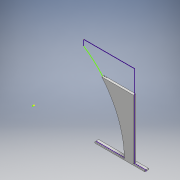
# Autodesk Inventor part: mtv_angle_2-2
Saved by Autodesk Inventor 2018 (Build 220112000, 112)
## iProperties
Created: 2019-02-03
Part Number: mtv_angle_2-2
Material: Generic
Document SubType Name: Modeling
Designer: Aditya Kendre
Density: 1 g/cm^3
Appearance: Default
Author: Aditya Kendre
## iProperties of the stored document mtv_angle_2-2_3DPrint.ipt
Created: 2019-02-03
Part Number: mtv_angle_2-2_3DPrint
Material: Generic
Document SubType Name: Modeling
Designer: Aditya Kendre
Density: 1 g/cm^3
Appearance: Default
Author: Aditya Kendre
Autodesk Inventor part; units mm, degrees
(part 1 of 2)
ref_plane "YZ Plane" through (0, 0, 0) normal (1, 0, 0) x (0, 1, 0)
ref_plane "XZ Plane" through (0, 0, 0) normal (0, 1, 0) x (-1, 0, 0)
ref_plane "XY Plane" through (0, 0, 0) normal (0, 0, 1) x (1, 0, 0)
sketch "Sketch1" plane through (0, 0, 0) normal (0, 1, 0) x (-1, 0, 0)
  line L0 (-225, -225) -> (225, -225)
  line L1 (225, -225) -> (225, 225)
  line L2 (225, 225) -> (-225, 225)
  line L3 (-225, 225) -> (-225, -225)
  line L4 (-225, -225) -> (225, 225) construction
  line L5 (225, -225) -> (-225, 225) construction
  point P0 (0, 0)
  dimension "d0" = 450
  dimension "d1" = 450
  constraints: 12 end point, 2 midpoint, 2 parallel, 1 horizontal, 1 perpendicular
  measures "d0" distance of L2.end L1.end
  measures "d1" distance of L1.end L0.end
extrude "Extrusion1" add sketch "Sketch1" along normal blind 3
sketch "Sketch2" plane through (0, 3, 0) normal (0, 1, 0) x (1, 0, 0)
  circle A0 centre (0, 0) radius 205
  dimension "d4" = 410
  constraints: 1 centre point, 1 coincident
  measures "d4" diameter of A0
extrude "Extrusion2" cut sketch "Sketch2" against normal blind 3
sketch "Sketch3" plane through (0, 3, 0) normal (0, 1, 0) x (1, 0, 0)
  circle A0 centre (0, 0) radius 205 projected
  line L0 (205, 0) -> (225, 0)
  line L1 (225, -225) -> (225, 225) projected
  line L2 (225, 0) -> (225, -225)
  line L3 (225, -225) -> (112.5, -225)
  line L4 (-225, -225) -> (225, -225) projected
  line L5 (112.5, -225) -> (112.5, 0)
  line L6 (112.5, 0) -> (225, 0)
  line L7 (112.5, -225) -> (-258.9889, -225)
  line L8 (-258.9889, -225) -> (-258.9889, 323.9574)
  line L9 (-258.9889, 323.9574) -> (112.5, 323.9574)
  line L10 (112.5, 323.9574) -> (112.5, -225)
  line L11 (225, 0) -> (-258.9889, 0)
  line L12 (-258.9889, 0) -> (-258.9889, 355.1924)
  line L13 (-258.9889, 355.1924) -> (225, 355.1924)
  line L14 (225, 355.1924) -> (225, 0)
  dimension "d7" = 112.5
  constraints: 26 end point, 4 parallel, 4 perpendicular, 3 point on line, 2 horizontal, 1 collinear, 1 horizontal alignment, 1 midpoint, 1 other
  measures "d7" distance of L1.start L3.end
extrude "Extrusion3" cut sketch "Sketch3" against normal blind 3 contours L6 L10 A0 | A0 L10 L9 L12 L13 L14 L1 L0 | L10 L11 A0 | A0 L11 L8 L9 L10 | L5 L4 L7 L8 L11 A0 | A0 L11 L5
sketch "Sketch4" plane through (0, 3, 0) normal (0, 1, 0) x (1, 0, 0)
  line L0 (112.5, -225) -> (225, -225) projected
  line L1 (225, -225) -> (225, 0) projected
  line L2 (112.5, -225) -> (225, -225)
  line L3 (225, -225) -> (225, -184.2834)
  line L4 (225, -184.2834) -> (112.5, -184.2834)
  line L5 (112.5, -184.2834) -> (112.5, -225)
  point P0 (0, 0)
  constraints: 8 end point, 2 parallel, 1 horizontal, 1 perpendicular, 1 point on line
extrude "Extrusion4" cut sketch "Sketch4" against normal blind 3
sketch "Sketch5" plane through (0, 3, 0) normal (0, 1, 0) x (1, 0, 0)
  line L0 (225, -184.2834) -> (225, 0) projected
  line L1 (225, 0) -> (140, 0)
  line L2 (140, 0) -> (140, -3)
  line L3 (140, -3) -> (225, -3)
  line L4 (225, -3) -> (225, 0)
  point P0 (0, 0)
  dimension "d12" = 85
  dimension "d13" = 3
  constraints: 8 end point, 2 parallel, 1 horizontal, 1 perpendicular
  measures "d12" distance of L3.end L2.end
  measures "d13" distance of L2.end L1.end
extrude "Extrusion5" add sketch "Sketch5" along normal mid plane 6
sketch "Sketch6" plane through (225, 0, 184.2834) normal (1, 0, 0) x (0, 0, -1)
  line L0 (181.2834, 3) -> (181.2834, 6) projected
  line L1 (184.2834, 0) -> (184.2834, 6) projected
  line L2 (181.2834, 6) -> (184.2834, 6)
  line L3 (184.2834, 6) -> (184.2834, 0)
  line L4 (184.2834, 0) -> (181.2834, 0)
  line L5 (181.2834, 0) -> (181.2834, 6)
  constraints: 8 end point, 2 parallel, 1 horizontal, 1 perpendicular
extrude "Extrusion6" add sketch "Sketch6" along normal blind 25
sketch "Sketch7" plane through (0, 3, 0) normal (0, 1, 0) x (1, 0, 0)
  arc A0 (112.5, -171.3731) -> (204.978, -3) centre (0, 0) ccw projected
  line L0 (204.978, -3) -> (140, -3) projected
  arc A1 (204.978, -3) -> (204.978, -3) centre (0, 0) ccw
  line L1 (112.5, -171.3731) -> (112.5, -173.3731)
  line L2 (112.5, -171.3731) -> (112.5, -184.2834) projected
  line L3 (204.978, -3) -> (206.978, -3)
  line L4 (140, -3) -> (250, -3) projected
  arc A2 (112.5, -173.3731) -> (206.978, -3) centre (3.682, -1.6473) ccw
  line L5 (206.1666, -3.9622) -> (206.1702, -3.6213)
  line L6 (206.1702, -3.6213) -> (210.1566, -3.6636)
  line L7 (210.1566, -3.6636) -> (210.153, -4.0044)
  line L8 (210.153, -4.0044) -> (206.1666, -3.9622)
  line L9 (206.1127, -6.8623) -> (206.1212, -6.5215)
  line L10 (206.1212, -6.5215) -> (210.1066, -6.6209)
  line L11 (210.1066, -6.6209) -> (210.0981, -6.9616)
  line L12 (210.0981, -6.9616) -> (206.1127, -6.8623)
  line L13 (206.0172, -9.7613) -> (206.0306, -9.4207)
  line L14 (206.0306, -9.4207) -> (210.0141, -9.5771)
  line L15 (210.0141, -9.5771) -> (210.0008, -9.9177)
  line L16 (210.0008, -9.9177) -> (206.0172, -9.7613)
  line L17 (205.8803, -12.6587) -> (205.8985, -12.3183)
  line L18 (205.8985, -12.3183) -> (209.8794, -12.5318)
  line L19 (209.8794, -12.5318) -> (209.8611, -12.8722)
  line L20 (209.8611, -12.8722) -> (205.8803, -12.6587)
  line L21 (205.7018, -15.5538) -> (205.7249, -15.2137)
  line L22 (205.7249, -15.2137) -> (209.7023, -15.4842)
  line L23 (209.7023, -15.4842) -> (209.6792, -15.8243)
  line L24 (209.6792, -15.8243) -> (205.7018, -15.5538)
  line L25 (205.4819, -18.4461) -> (205.5099, -18.1064)
  line L26 (205.5099, -18.1064) -> (209.483, -18.4338)
  line L27 (209.483, -18.4338) -> (209.455, -18.7735)
  line L28 (209.455, -18.7735) -> (205.4819, -18.4461)
  line L29 (205.2205, -21.3349) -> (205.2534, -20.9956)
  line L30 (205.2534, -20.9956) -> (209.2214, -21.3799)
  line L31 (209.2214, -21.3799) -> (209.1886, -21.7192)
  line L32 (209.1886, -21.7192) -> (205.2205, -21.3349)
  line L33 (204.9179, -24.2197) -> (204.9556, -23.8809)
  line L34 (204.9556, -23.8809) -> (208.9177, -24.322)
  line L35 (208.9177, -24.322) -> (208.88, -24.6608)
  line L36 (208.88, -24.6608) -> (204.9179, -24.2197)
  line L37 (204.5739, -27.0998) -> (204.6165, -26.7616)
  line L38 (204.6165, -26.7616) -> (208.5719, -27.2594)
  line L39 (208.5719, -27.2594) -> (208.5293, -27.5976)
  line L40 (208.5293, -27.5976) -> (204.5739, -27.0998)
  line L41 (204.1887, -29.9747) -> (204.2361, -29.6372)
  line L42 (204.2361, -29.6372) -> (208.184, -30.1916)
  line L43 (208.184, -30.1916) -> (208.1366, -30.5291)
  line L44 (208.1366, -30.5291) -> (204.1887, -29.9747)
  line L45 (203.7624, -32.8439) -> (203.8146, -32.507)
  line L46 (203.8146, -32.507) -> (207.7541, -33.1179)
  line L47 (207.7541, -33.1179) -> (207.7019, -33.4547)
  line L48 (207.7019, -33.4547) -> (203.7624, -32.8439)
  line L49 (203.295, -35.7066) -> (203.3521, -35.3705)
  line L50 (203.3521, -35.3705) -> (207.2824, -36.0378)
  line L51 (207.2824, -36.0378) -> (207.2254, -36.3738)
  line L52 (207.2254, -36.3738) -> (203.295, -35.7066)
  line L53 (202.7867, -38.5623) -> (202.8485, -38.2271)
  line L54 (202.8485, -38.2271) -> (206.7689, -38.9506)
  line L55 (206.7689, -38.9506) -> (206.7071, -39.2858)
  line L56 (206.7071, -39.2858) -> (202.7867, -38.5623)
  line L57 (202.2375, -41.4104) -> (202.3041, -41.0762)
  line L58 (202.3041, -41.0762) -> (206.2138, -41.8557)
  line L59 (206.2138, -41.8557) -> (206.1471, -42.19)
  line L60 (206.1471, -42.19) -> (202.2375, -41.4104)
  line L61 (201.6476, -44.2504) -> (201.719, -43.9171)
  line L62 (201.719, -43.9171) -> (205.6171, -44.7526)
  line L63 (205.6171, -44.7526) -> (205.5456, -45.0859)
  line L64 (205.5456, -45.0859) -> (201.6476, -44.2504)
  line L65 (201.017, -47.0817) -> (201.0932, -46.7494)
  line L66 (201.0932, -46.7494) -> (204.9789, -47.6407)
  line L67 (204.9789, -47.6407) -> (204.9027, -47.9729)
  line L68 (204.9027, -47.9729) -> (201.017, -47.0817)
  line L69 (200.346, -49.9036) -> (200.4269, -49.5725)
  line L70 (200.4269, -49.5725) -> (204.2995, -50.5193)
  line L71 (204.2995, -50.5193) -> (204.2185, -50.8504)
  line L72 (204.2185, -50.8504) -> (200.346, -49.9036)
  line L73 (199.6346, -52.7156) -> (199.7203, -52.3857)
  line L74 (199.7203, -52.3857) -> (203.5789, -53.3879)
  line L75 (203.5789, -53.3879) -> (203.4932, -53.7178)
  line L76 (203.4932, -53.7178) -> (199.6346, -52.7156)
  line L77 (198.883, -55.5172) -> (198.9734, -55.1885)
  line L78 (198.9734, -55.1885) -> (202.8172, -56.2459)
  line L79 (202.8172, -56.2459) -> (202.7268, -56.5745)
  line L80 (202.7268, -56.5745) -> (198.883, -55.5172)
  line L81 (198.0913, -58.3077) -> (198.1864, -57.9803)
  line L82 (198.1864, -57.9803) -> (202.0147, -59.0926)
  line L83 (202.0147, -59.0926) -> (201.9196, -59.42)
  line L84 (201.9196, -59.42) -> (198.0913, -58.3077)
  line L85 (197.2598, -61.0865) -> (197.3596, -60.7606)
  line L86 (197.3596, -60.7606) -> (201.1716, -61.9276)
  line L87 (201.1716, -61.9276) -> (201.0718, -62.2535)
  line L88 (201.0718, -62.2535) -> (197.2598, -61.0865)
  line L89 (196.3885, -63.8532) -> (196.493, -63.5287)
  line L90 (196.493, -63.5287) -> (200.2879, -64.7502)
  line L91 (200.2879, -64.7502) -> (200.1834, -65.0747)
  line L92 (200.1834, -65.0747) -> (196.3885, -63.8532)
  line L93 (195.4778, -66.6071) -> (195.5868, -66.2842)
  line L94 (195.5868, -66.2842) -> (199.3638, -67.5599)
  line L95 (199.3638, -67.5599) -> (199.2547, -67.8828)
  line L96 (199.2547, -67.8828) -> (195.4778, -66.6071)
  line L97 (194.5276, -69.3477) -> (194.6413, -69.0264)
  line L98 (194.6413, -69.0264) -> (198.3996, -70.356)
  line L99 (198.3996, -70.356) -> (198.2859, -70.6774)
  line L100 (198.2859, -70.6774) -> (194.5276, -69.3477)
  line L101 (193.5383, -72.0744) -> (193.6566, -71.7547)
  line L102 (193.6566, -71.7547) -> (197.3955, -73.1381)
  line L103 (197.3955, -73.1381) -> (197.2772, -73.4578)
  line L104 (197.2772, -73.4578) -> (193.5383, -72.0744)
  line L105 (192.51, -74.7866) -> (192.6329, -74.4687)
  line L106 (192.6329, -74.4687) -> (196.3516, -75.9055)
  line L107 (196.3516, -75.9055) -> (196.2287, -76.2234)
  line L108 (196.2287, -76.2234) -> (192.51, -74.7866)
  line L109 (191.443, -77.4839) -> (191.5704, -77.1677)
  line L110 (191.5704, -77.1677) -> (195.2681, -78.6576)
  line L111 (195.2681, -78.6576) -> (195.1408, -78.9738)
  line L112 (195.1408, -78.9738) -> (191.443, -77.4839)
  line L113 (190.3375, -80.1655) -> (190.4694, -79.8512)
  line L114 (190.4694, -79.8512) -> (194.1454, -81.394)
  line L115 (194.1454, -81.394) -> (194.0135, -81.7083)
  line L116 (194.0135, -81.7083) -> (190.3375, -80.1655)
  line L117 (189.1937, -82.8311) -> (189.3301, -82.5187)
  line L118 (189.3301, -82.5187) -> (192.9836, -84.1139)
  line L119 (192.9836, -84.1139) -> (192.8472, -84.4263)
  line L120 (192.8472, -84.4263) -> (189.1937, -82.8311)
  line L121 (188.0118, -85.48) -> (188.1526, -85.1696)
  line L122 (188.1526, -85.1696) -> (191.7829, -86.817)
  line L123 (191.7829, -86.817) -> (191.6421, -87.1274)
  line L124 (191.6421, -87.1274) -> (188.0118, -85.48)
  line L125 (186.7921, -88.1117) -> (186.9374, -87.8034)
  line L126 (186.9374, -87.8034) -> (190.5437, -89.5026)
  line L127 (190.5437, -89.5026) -> (190.3984, -89.8109)
  line L128 (190.3984, -89.8109) -> (186.7921, -88.1117)
  line L129 (185.5348, -90.7257) -> (185.6845, -90.4194)
  line L130 (185.6845, -90.4194) -> (189.2661, -92.1701)
  line L131 (189.2661, -92.1701) -> (189.1164, -92.4764)
  line L132 (189.1164, -92.4764) -> (185.5348, -90.7257)
  line L133 (184.2402, -93.3213) -> (184.3942, -93.0173)
  line L134 (184.3942, -93.0173) -> (187.9504, -94.8191)
  line L135 (187.9504, -94.8191) -> (187.7964, -95.1232)
  line L136 (187.7964, -95.1232) -> (184.2402, -93.3213)
  line L137 (182.9085, -95.8982) -> (183.0669, -95.5964)
  line L138 (183.0669, -95.5964) -> (186.597, -97.449)
  line L139 (186.597, -97.449) -> (186.4386, -97.7508)
  line L140 (186.4386, -97.7508) -> (182.9085, -95.8982)
  line L141 (181.5401, -98.4558) -> (181.7028, -98.1562)
  line L142 (181.7028, -98.1562) -> (185.2059, -100.0592)
  line L143 (185.2059, -100.0592) -> (185.0432, -100.3587)
  line L144 (185.0432, -100.3587) -> (181.5401, -98.4558)
  line L145 (180.1352, -100.9934) -> (180.3022, -100.6963)
  line L146 (180.3022, -100.6963) -> (183.7777, -102.6492)
  line L147 (183.7777, -102.6492) -> (183.6107, -102.9464)
  line L148 (183.6107, -102.9464) -> (180.1352, -100.9934)
  line L149 (178.6941, -103.5107) -> (178.8653, -103.216)
  line L150 (178.8653, -103.216) -> (182.3125, -105.2185)
  line L151 (182.3125, -105.2185) -> (182.1413, -105.5132)
  line L152 (182.1413, -105.5132) -> (178.6941, -103.5107)
  line L153 (177.2171, -106.0071) -> (177.3925, -105.7149)
  line L154 (177.3925, -105.7149) -> (180.8106, -107.7665)
  line L155 (180.8106, -107.7665) -> (180.6352, -108.0588)
  line L156 (180.6352, -108.0588) -> (177.2171, -106.0071)
  line L157 (175.7044, -108.4821) -> (175.884, -108.1924)
  line L158 (175.884, -108.1924) -> (179.2724, -110.2928)
  line L159 (179.2724, -110.2928) -> (179.0928, -110.5825)
  line L160 (179.0928, -110.5825) -> (175.7044, -108.4821)
  line L161 (174.1565, -110.9351) -> (174.3402, -110.648)
  line L162 (174.3402, -110.648) -> (177.6982, -112.7968)
  line L163 (177.6982, -112.7968) -> (177.5145, -113.0839)
  line L164 (177.5145, -113.0839) -> (174.1565, -110.9351)
  line L165 (172.5736, -113.3658) -> (172.7614, -113.0813)
  line L166 (172.7614, -113.0813) -> (176.0883, -115.278)
  line L167 (176.0883, -115.278) -> (175.9004, -115.5624)
  line L168 (175.9004, -115.5624) -> (172.5736, -113.3658)
  line L169 (170.956, -115.7735) -> (171.1479, -115.4917)
  line L170 (171.1479, -115.4917) -> (174.4429, -117.7358)
  line L171 (174.4429, -117.7358) -> (174.2511, -118.0175)
  line L172 (174.2511, -118.0175) -> (170.956, -115.7735)
  line L173 (169.3042, -118.1578) -> (169.5001, -117.8788)
  line L174 (169.5001, -117.8788) -> (172.7626, -120.1698)
  line L175 (172.7626, -120.1698) -> (172.5667, -120.4488)
  line L176 (172.5667, -120.4488) -> (169.3042, -118.1578)
  line L177 (167.6183, -120.5182) -> (167.8182, -120.242)
  line L178 (167.8182, -120.242) -> (171.0476, -122.5796)
  line L179 (171.0476, -122.5796) -> (170.8477, -122.8557)
  line L180 (170.8477, -122.8557) -> (167.6183, -120.5182)
  line L181 (165.8988, -122.8542) -> (166.1026, -122.5809)
  line L182 (166.1026, -122.5809) -> (169.2982, -124.9645)
  line L183 (169.2982, -124.9645) -> (169.0944, -125.2377)
  line L184 (169.0944, -125.2377) -> (165.8988, -122.8542)
  line L185 (164.146, -125.1653) -> (164.3537, -124.895)
  line L186 (164.3537, -124.895) -> (167.5148, -127.3241)
  line L187 (167.5148, -127.3241) -> (167.3071, -127.5944)
  line L188 (167.3071, -127.5944) -> (164.146, -125.1653)
  line L189 (162.3603, -127.4511) -> (162.5718, -127.1838)
  line L190 (162.5718, -127.1838) -> (165.6978, -129.6579)
  line L191 (165.6978, -129.6579) -> (165.4863, -129.9252)
  line L192 (165.4863, -129.9252) -> (162.3603, -127.4511)
  line L193 (160.542, -129.711) -> (160.7574, -129.4468)
  line L194 (160.7574, -129.4468) -> (163.8476, -131.9654)
  line L195 (163.8476, -131.9654) -> (163.6323, -132.2297)
  line L196 (163.6323, -132.2297) -> (160.542, -129.711)
  line L197 (158.6916, -131.9447) -> (158.9107, -131.6836)
  line L198 (158.9107, -131.6836) -> (161.9645, -134.2462)
  line L199 (161.9645, -134.2462) -> (161.7454, -134.5074)
  line L200 (161.7454, -134.5074) -> (158.6916, -131.9447)
  line L201 (156.8093, -134.1517) -> (157.0322, -133.8937)
  line L202 (157.0322, -133.8937) -> (160.049, -136.4999)
  line L203 (160.049, -136.4999) -> (159.8261, -136.7578)
  line L204 (159.8261, -136.7578) -> (156.8093, -134.1517)
  line L205 (154.8957, -136.3315) -> (155.1222, -136.0767)
  line L206 (155.1222, -136.0767) -> (158.1013, -138.7258)
  line L207 (158.1013, -138.7258) -> (157.8748, -138.9805)
  line L208 (157.8748, -138.9805) -> (154.8957, -136.3315)
  line L209 (152.951, -138.4836) -> (153.1811, -138.2321)
  line L210 (153.1811, -138.2321) -> (156.122, -140.9236)
  line L211 (156.122, -140.9236) -> (155.8919, -141.1751)
  line L212 (155.8919, -141.1751) -> (152.951, -138.4836)
  line L213 (150.9756, -140.6077) -> (151.2093, -140.3595)
  line L214 (151.2093, -140.3595) -> (154.1114, -143.0928)
  line L215 (154.1114, -143.0928) -> (153.8777, -143.341)
  line L216 (153.8777, -143.341) -> (150.9756, -140.6077)
  line L217 (148.9701, -142.7032) -> (149.2073, -142.4584)
  line L218 (149.2073, -142.4584) -> (152.0699, -145.233)
  line L219 (152.0699, -145.233) -> (151.8327, -145.4778)
  line L220 (151.8327, -145.4778) -> (148.9701, -142.7032)
  line L221 (146.9347, -144.7698) -> (147.1754, -144.5285)
  line L222 (147.1754, -144.5285) -> (149.998, -147.3438)
  line L223 (149.998, -147.3438) -> (149.7573, -147.5851)
  line L224 (149.7573, -147.5851) -> (146.9347, -144.7698)
  line L225 (144.87, -146.807) -> (145.1141, -146.5692)
  line L226 (145.1141, -146.5692) -> (147.8961, -149.4246)
  line L227 (147.8961, -149.4246) -> (147.6519, -149.6625)
  line L228 (147.6519, -149.6625) -> (144.87, -146.807)
  line L229 (142.7762, -148.8145) -> (143.0238, -148.5802)
  line L230 (143.0238, -148.5802) -> (145.7645, -151.4752)
  line L231 (145.7645, -151.4752) -> (145.517, -151.7095)
  line L232 (145.517, -151.7095) -> (142.7762, -148.8145)
  line L233 (140.654, -150.7918) -> (140.9048, -150.561)
  line L234 (140.9048, -150.561) -> (143.6039, -153.495)
  line L235 (143.6039, -153.495) -> (143.353, -153.7257)
  line L236 (143.353, -153.7257) -> (140.654, -150.7918)
  line L237 (138.5036, -152.7384) -> (138.7577, -152.5113)
  line L238 (138.7577, -152.5113) -> (141.4145, -155.4836)
  line L239 (141.4145, -155.4836) -> (141.1603, -155.7108)
  line L240 (141.1603, -155.7108) -> (138.5036, -152.7384)
  line L241 (136.3256, -154.6541) -> (136.5829, -154.4306)
  line L242 (136.5829, -154.4306) -> (139.1968, -157.4407)
  line L243 (139.1968, -157.4407) -> (138.9395, -157.6642)
  line L244 (138.9395, -157.6642) -> (136.3256, -154.6541)
  line L245 (134.1203, -156.5383) -> (134.3809, -156.3186)
  line L246 (134.3809, -156.3186) -> (136.9514, -159.3658)
  line L247 (136.9514, -159.3658) -> (136.6908, -159.5856)
  line L248 (136.6908, -159.5856) -> (134.1203, -156.5383)
  line L249 (131.8883, -158.3908) -> (132.152, -158.1748)
  line L250 (132.152, -158.1748) -> (134.6786, -161.2585)
  line L251 (134.6786, -161.2585) -> (134.4149, -161.4745)
  line L252 (134.4149, -161.4745) -> (131.8883, -158.3908)
  line L253 (129.63, -160.2111) -> (129.8967, -159.9989)
  line L254 (129.8967, -159.9989) -> (132.3789, -163.1185)
  line L255 (132.3789, -163.1185) -> (132.1122, -163.3307)
  line L256 (132.1122, -163.3307) -> (129.63, -160.2111)
  line L257 (127.3458, -161.9989) -> (127.6156, -161.7905)
  line L258 (127.6156, -161.7905) -> (130.0528, -164.9454)
  line L259 (130.0528, -164.9454) -> (129.7831, -165.1538)
  line L260 (129.7831, -165.1538) -> (127.3458, -161.9989)
  line L261 (125.0363, -163.7538) -> (125.309, -163.5493)
  line L262 (125.309, -163.5493) -> (127.7008, -166.7387)
  line L263 (127.7008, -166.7387) -> (127.4281, -166.9432)
  line L264 (127.4281, -166.9432) -> (125.0363, -163.7538)
  line L265 (122.7019, -165.4754) -> (122.9775, -165.2749)
  line L266 (122.9775, -165.2749) -> (125.3233, -168.4982)
  line L267 (125.3233, -168.4982) -> (125.0477, -168.6988)
  line L268 (125.0477, -168.6988) -> (122.7019, -165.4754)
  line L269 (120.343, -167.1635) -> (120.6215, -166.9668)
  line L270 (120.6215, -166.9668) -> (122.9209, -170.2235)
  line L271 (122.9209, -170.2235) -> (122.6425, -170.4201)
  line L272 (122.6425, -170.4201) -> (120.343, -167.1635)
  line L273 (117.9602, -168.8175) -> (118.2415, -168.6249)
  line L274 (118.2415, -168.6249) -> (120.494, -171.9141)
  line L275 (120.494, -171.9141) -> (120.2128, -172.1067)
  line L276 (120.2128, -172.1067) -> (117.9602, -168.8175)
  line L277 (115.554, -170.4372) -> (115.838, -170.2487)
  line L278 (115.838, -170.2487) -> (118.0432, -173.5698)
  line L279 (118.0432, -173.5698) -> (117.7592, -173.7584)
  line L280 (117.7592, -173.7584) -> (115.554, -170.4372)
  line L281 (113.1248, -172.0224) -> (113.4114, -171.8379)
  line L282 (113.4114, -171.8379) -> (115.5689, -175.1903)
  line L283 (115.5689, -175.1903) -> (115.2822, -175.3748)
  line L284 (115.2822, -175.3748) -> (113.1248, -172.0224)
  dimension "d18" = 2
  dimension "d19" = 2
  constraints: 4 end point, 2 point on circle, 2 point on line, 1 centre point, 5 other
  measures "d18" distance of L1.start L1.end
  measures "d19" distance of L0.start L3.end
emboss "Emboss1" sketch "Sketch7" operation cut depth 2 direction (0, -1, 0) contours L284 L281 L282 A2 | A2 L282 L283 L284 | L6 L7 L8 A2 | A2 L8 L5 L6 | L280 L277 L278 A2 | A2 L278 L279 L280 | L10 L11 L12 A2 | A2 L12 L9 L10 | L276 L273 L274 A2 | A2 L274 L275 L276 | L14 L15 L16 A2 | A2 L16 L13 L14 | L272 L269 L270 A2 | A2 L270 L271 L272 | L18 L19 L20 A2 | A2 L20 L17 L18 | L268 L265 L266 A2 | A2 L266 L267 L268 | L22 L23 L24 A2 | A2 L24 L21 L22 | L264 L261 L262 A2 | A2 L262 L263 L264 | L26 L27 L28 A2 | A2 L28 L25 L26 | L260 L257 L258 A2 | A2 L258 L259 L260 | L30 L31 L32 A2 | A2 L32 L29 L30 | L256 L253 L254 A2 | A2 L254 L255 L256 | L34 L35 L36 A2 | A2 L36 L33 L34 | L252 L249 L250 A2 | A2 L250 L251 L252 | L38 L39 L40 A2 | A2 L40 L37 L38 | L248 L245 L246 A2 | A2 L246 L247 L248 | L42 L43 L44 A2 | A2 L44 L41 L42 | L244 L241 L242 A2 | A2 L242 L243 L244 | L46 L47 L48 A2 | A2 L48 L45 L46 | L240 L237 L238 A2 | A2 L238 L239 L240 | L50 L51 L52 A2 | A2 L52 L49 L50 | L236 L233 L234 A2 | A2 L234 L235 L236 | L54 L55 L56 A2 | A2 L56 L53 L54 | L232 L229 L230 A2 | A2 L230 L231 L232 | L58 L59 L60 A2 | A2 L60 L57 L58 | L228 L225 L226 A2 | A2 L226 L227 L228 | L62 L63 L64 A2 | A2 L64 L61 L62 | L224 L221 L222 A2 | A2 L222 L223 L224 | L66 L67 L68 A2 | A2 L68 L65 L66 | L220 L217 L218 A2 | A2 L218 L219 L220 | L70 L71 L72 A2 | A2 L72 L69 L70 | L216 L213 L214 A2 | A2 L214 L215 L216 | L74 L75 L76 A2 | A2 L76 L73 L74 | L212 L209 L210 A2 | A2 L210 L211 L212 | L78 L79 L80 A2 | A2 L80 L77 L78 | L208 L205 L206 A2 | A2 L206 L207 L208 | L82 L83 L84 A2 | A2 L84 L81 L82 | L204 L201 L202 A2 | A2 L202 L203 L204 | L86 L87 L88 A2 | A2 L88 L85 L86 | L200 L197 L198 A2 | A2 L198 L199 L200 | L90 L91 L92 A2 | A2 L92 L89 L90 | L196 L193 L194 A2 | A2 L194 L195 L196 | L94 L95 L96 A2 | A2 L96 L93 L94 | L192 L189 L190 A2 | A2 L190 L191 L192 | L98 L99 L100 A2 | A2 L100 L97 L98 | L188 L185 L186 A2 | A2 L186 L187 L188 | L102 L103 L104 A2 | A2 L104 L101 L102 | L184 L181 L182 A2 | A2 L182 L183 L184 | L106 L107 L108 A2 | A2 L108 L105 L106 | L180 L177 L178 A2 | A2 L178 L179 L180 | L110 L111 L112 A2 | A2 L112 L109 L110 | L176 L173 L174 A2 | A2 L174 L175 L176 | L114 L115 L116 A2 | A2 L116 L113 L114 | L172 L169 L170 A2 | A2 L170 L171 L172 | L118 L119 L120 A2 | A2 L120 L117 L118 | L168 L165 L166 A2 | A2 L166 L167 L168 | L122 L123 L124 A2 | A2 L124 L121 L122 | L164 L161 L162 A2 | A2 L162 L163 L164 | L126 L127 L128 A2 | A2 L128 L125 L126 | L160 L157 L158 A2 | A2 L158 L159 L160 | L130 L131 L132 A2 | A2 L132 L129 L130 | L156 L153 L154 A2 | A2 L154 L155 L156 | L134 L135 L136 A2 | A2 L136 L133 L134 | L152 L149 L150 A2 | A2 L150 L151 L152 | L138 L139 L140 A2 | A2 L140 L137 L138 | L148 L145 L146 A2 | A2 L146 L147 L148 | L142 L143 L144 A2 | A2 L144 L141 L142
sketch "Sketch8" plane through (0, 0, 0) normal (0, -1, 0) x (1, 0, 0)
  line L0 (140, 0) -> (250, 0) projected
  line L1 (225, 3) -> (250, 3) projected
  line L2 (140, 0) -> (250, 0)
  line L3 (250, 0) -> (250, 3)
  line L4 (250, 3) -> (140, 3)
  line L5 (140, 3) -> (140, 0)
  arc A0 (204.978, 3) -> (112.5, 171.3731) centre (0, 0) ccw projected
  arc A1 (204.978, 3) -> (112.5, 171.3731) centre (0, 0) ccw
  line L6 (225, 184.2834) -> (225, 3) projected
  line L7 (225, 3) -> (225, 184.2834)
  line L8 (112.5, 184.2834) -> (225, 184.2834) projected
  line L9 (225, 184.2834) -> (112.5, 184.2834)
  line L10 (112.5, 184.2834) -> (112.5, 171.3731)
  constraints: 14 end point, 3 perpendicular, 2 parallel, 2 point on circle, 1 centre point, 1 horizontal, 1 vertical
sketch "Sketch9" plane through (0, 0, 0) normal (0, -1, 0) x (1, 0, 0)
  line L0 (204.978, 3) -> (140, 3) projected
  line L1 (204.978, 3) -> (225, 3)
  point P0 (0, 0)
  constraints: 2 end point, 1 horizontal
sketch "Sketch10" plane through (0, 0, 0) normal (0, -1, 0) x (1, 0, 0)
  line L0 (140, 0) -> (250, 0) projected
  line L1 (225, 3) -> (250, 3) projected
  line L2 (140, 0) -> (250, 0)
  line L3 (250, 0) -> (250, 3)
  line L4 (250, 3) -> (140, 3)
  line L5 (140, 3) -> (140, 0)
  line L6 (204.978, 3) -> (140, 3) projected
  line L7 (112.5, 171.3731) -> (112.5, 184.2834) projected
  arc A0 (204.978, 3) -> (112.5, 171.3731) centre (0, 0) ccw
  line L8 (112.5, 171.3731) -> (112.5, 184.2834)
  line L9 (225, 184.2834) -> (225, 3) projected
  line L10 (112.5, 184.2834) -> (225, 184.2834) projected
  line L11 (225, 184.2834) -> (112.5, 184.2834)
  line L12 (112.5, 184.2834) -> (225, 184.2834)
  line L13 (225, 3) -> (225, 184.2834)
  line L14 (204.978, 3) -> (225, 3)
  point P0 (0, 0)
  constraints: 18 end point, 3 collinear, 2 horizontal, 2 parallel, 2 perpendicular, 2 point on circle, 1 centre point
extrude "Extrusion7" add sketch "Sketch10" along normal blind 2
sketch "Sketch11" plane through (0, 3, 0) normal (0, 1, 0) x (1, 0, 0)
  line L0 (112.5, -171.3731) -> (112.5, -178.3731)
  line L1 (112.5, -171.3731) -> (112.5, -184.2834) projected
  arc A0 (112.5, -171.3731) -> (204.978, -3) centre (0, 0) ccw projected
  line L2 (140, -3) -> (250, -3) projected
  arc A1 (112.5, -178.3731) -> (211.978, -3) centre (9.6426, -4.1283) ccw
  spline S0 degree 2 poles (212.18, -4.2741) (212.1516, -4.2356) (212.0502, -4.1061) (212.0197, -4.0453) knots 0 0 0 1 2 2 2
  spline S1 degree 2 poles (212.0197, -4.0453) (211.9751, -3.9623) (211.9283, -3.8064) (211.9281, -3.6646) knots 0 0 0 1 2 2 2
  spline S2 degree 2 poles (211.9281, -3.6646) (211.928, -3.5491) (212.0149, -3.3403) (212.0938, -3.2612) knots 0 0 0 1 2 2 2
  spline S3 degree 2 poles (212.0938, -3.2612) (212.1707, -3.1862) (212.3975, -3.0947) (212.5231, -3.0946) knots 0 0 0 1 2 2 2
  spline S4 degree 2 poles (212.5231, -3.0946) (212.7176, -3.0944) (212.9933, -3.2582) (213.0725, -3.4364) knots 0 0 0 1 2 2 2
  spline S5 degree 2 poles (213.0725, -3.4364) (213.1456, -3.5943) (213.2008, -4.0237) (213.2153, -4.2729) knots 0 0 0 1 2 2 2
  line L3 (213.2153, -4.2729) -> (213.2761, -4.2729)
  spline S6 degree 2 poles (213.2761, -4.2729) (213.3855, -4.2727) (213.5211, -4.2057) (213.5595, -4.1449) knots 0 0 0 1 2 2 2
  spline S7 degree 2 poles (213.5595, -4.1449) (213.598, -4.0841) (213.6221, -3.9098) (213.622, -3.8166) knots 0 0 0 1 2 2 2
  spline S8 degree 2 poles (213.622, -3.8166) (213.6219, -3.7072) (213.5567, -3.4115) (213.4937, -3.2637) knots 0 0 0 1 2 2 2
  line L4 (213.4937, -3.2637) -> (213.4937, -3.2455)
  line L5 (213.4937, -3.2455) -> (213.8158, -3.2451)
  spline S9 degree 2 poles (213.8158, -3.2451) (213.8402, -3.3322) (213.9014, -3.6583) (213.9016, -3.8183) knots 0 0 0 1 2 2 2
  spline S10 degree 2 poles (213.9016, -3.8183) (213.9018, -4.0128) (213.8413, -4.2783) (213.7624, -4.3837) knots 0 0 0 1 2 2 2
  spline S11 degree 2 poles (213.7624, -4.3837) (213.6855, -4.4871) (213.4405, -4.5887) (213.2642, -4.5889) knots 0 0 0 1 2 2 2
  line L6 (213.2642, -4.5889) -> (211.9818, -4.5903)
  line L7 (211.9818, -4.5903) -> (211.9815, -4.2743)
  line L8 (211.9815, -4.2743) -> (212.18, -4.2741)
  line L9 (212.4434, -4.2738) -> (212.9641, -4.2732)
  spline S12 degree 2 poles (212.9641, -4.2732) (212.9538, -4.1598) (212.919, -3.8174) (212.8864, -3.7101) knots 0 0 0 1 2 2 2
  spline S13 degree 2 poles (212.8864, -3.7101) (212.8478, -3.5845) (212.6876, -3.4206) (212.5458, -3.4208) knots 0 0 0 1 2 2 2
  spline S14 degree 2 poles (212.5458, -3.4208) (212.3837, -3.4209) (212.2198, -3.6034) (212.22, -3.7777) knots 0 0 0 1 2 2 2
  spline S15 degree 2 poles (212.22, -3.7777) (212.2202, -3.9256) (212.3481, -4.1685) (212.4434, -4.2738) knots 0 0 0 1 2 2 2
  spline S16 degree 2 poles (212.9201, -7.6926) (212.4603, -7.6865) (211.9051, -7.2334) (211.9096, -6.8971) knots 0 0 0 1 2 2 2
  spline S17 degree 2 poles (211.9096, -6.8971) (211.9116, -6.7451) (211.9895, -6.5294) (212.0557, -6.4249) knots 0 0 0 1 2 2 2
  line L10 (212.0557, -6.4249) -> (211.9688, -6.4035)
  line L11 (211.9688, -6.4035) -> (211.9728, -6.1077)
  line L12 (211.9728, -6.1077) -> (214.584, -6.1426)
  line L13 (214.584, -6.1426) -> (214.5798, -6.4586)
  line L14 (214.5798, -6.4586) -> (213.6479, -6.4462)
  spline S18 degree 2 poles (213.6479, -6.4462) (213.7537, -6.5671) (213.8918, -6.8465) (213.8894, -7.0228) knots 0 0 0 1 2 2 2
  spline S19 degree 2 poles (213.8894, -7.0228) (213.8852, -7.3408) (213.3719, -7.6987) (212.9201, -7.6926) knots 0 0 0 1 2 2 2
  spline S20 degree 2 poles (212.9002, -7.3662) (213.2364, -7.3707) (213.5876, -7.1707) (213.5906, -6.9438) knots 0 0 0 1 2 2 2
  spline S21 degree 2 poles (213.5906, -6.9438) (213.5923, -6.8162) (213.4743, -6.5512) (213.3826, -6.4426) knots 0 0 0 1 2 2 2
  line L15 (213.3826, -6.4426) -> (212.3069, -6.4283)
  spline S22 degree 2 poles (212.3069, -6.4283) (212.2465, -6.547) (212.1955, -6.7307) (212.194, -6.8401) knots 0 0 0 1 2 2 2
  spline S23 degree 2 poles (212.194, -6.8401) (212.1908, -7.0812) (212.5295, -7.3612) (212.9002, -7.3662) knots 0 0 0 1 2 2 2
  spline S24 degree 2 poles (211.8585, -9.8254) (211.8638, -9.631) (211.9921, -9.3123) (212.1167, -9.2002) knots 0 0 0 1 2 2 2
  spline S25 degree 2 poles (212.1167, -9.2002) (212.2394, -9.088) (212.6114, -8.9704) (212.8585, -8.9772) knots 0 0 0 1 2 2 2
  spline S26 degree 2 poles (212.8585, -8.9772) (213.1056, -8.9839) (213.4625, -9.1254) (213.5809, -9.2401) knots 0 0 0 1 2 2 2
  spline S27 degree 2 poles (213.5809, -9.2401) (213.7014, -9.3548) (213.8241, -9.6885) (213.8189, -9.8789) knots 0 0 0 1 2 2 2
  spline S28 degree 2 poles (213.8189, -9.8789) (213.8147, -10.0328) (213.7197, -10.318) (213.66, -10.4279) knots 0 0 0 1 2 2 2
  line L16 (213.66, -10.4279) -> (213.3056, -10.4182)
  line L17 (213.3056, -10.4182) -> (213.3061, -10.4)
  spline S29 degree 2 poles (213.3061, -10.4) (213.3354, -10.3663) (213.4112, -10.263) (213.4517, -10.1891) knots 0 0 0 1 2 2 2
  spline S30 degree 2 poles (213.4517, -10.1891) (213.4859, -10.1232) (213.5414, -9.9463) (213.5436, -9.8653) knots 0 0 0 1 2 2 2
  spline S31 degree 2 poles (213.5436, -9.8653) (213.5503, -9.6203) (213.1878, -9.3125) (212.8496, -9.3032) knots 0 0 0 1 2 2 2
  spline S32 degree 2 poles (212.8496, -9.3032) (212.5195, -9.2942) (212.141, -9.5717) (212.1341, -9.8269) knots 0 0 0 1 2 2 2
  spline S33 degree 2 poles (212.1341, -9.8269) (212.1299, -9.9808) (212.2498, -10.2637) (212.3462, -10.3738) knots 0 0 0 1 2 2 2
  line L18 (212.3462, -10.3738) -> (212.3457, -10.392)
  line L19 (212.3457, -10.392) -> (211.9913, -10.3823)
  spline S34 degree 2 poles (211.9913, -10.3823) (211.9702, -10.3352) (211.9113, -10.1917) (211.8987, -10.1346) knots 0 0 0 1 2 2 2
  spline S35 degree 2 poles (211.8987, -10.1346) (211.8766, -10.0529) (211.8558, -9.9247) (211.8585, -9.8254) knots 0 0 0 1 2 2 2
  line L20 (211.7799, -13.1813) -> (211.7929, -12.8656)
  line L21 (211.7929, -12.8656) -> (211.9831, -12.8734)
  spline S36 degree 2 poles (211.9831, -12.8734) (211.9254, -12.798) (211.8489, -12.6874) (211.8175, -12.6131) knots 0 0 0 1 2 2 2
  spline S37 degree 2 poles (211.8175, -12.6131) (211.7878, -12.545) (211.7593, -12.3998) (211.7633, -12.3047) knots 0 0 0 1 2 2 2
  spline S38 degree 2 poles (211.7633, -12.3047) (211.7696, -12.1509) (211.9078, -11.897) (212.035, -11.811) knots 0 0 0 1 2 2 2
  spline S39 degree 2 poles (212.035, -11.811) (212.1623, -11.725) (212.5308, -11.6388) (212.7676, -11.6486) knots 0 0 0 1 2 2 2
  spline S40 degree 2 poles (212.7676, -11.6486) (213.0146, -11.6588) (213.3696, -11.8011) (213.5007, -11.9181) knots 0 0 0 1 2 2 2
  spline S41 degree 2 poles (213.5007, -11.9181) (213.6179, -12.0263) (213.7456, -12.3215) (213.739, -12.4814) knots 0 0 0 1 2 2 2
  spline S42 degree 2 poles (213.739, -12.4814) (213.7333, -12.6211) (213.6619, -12.827) (213.5924, -12.9397) knots 0 0 0 1 2 2 2
  line L22 (213.5924, -12.9397) -> (214.4021, -12.9731)
  line L23 (214.4021, -12.9731) -> (214.3891, -13.2889)
  line L24 (214.3891, -13.2889) -> (211.7799, -13.1813)
  line L25 (212.2483, -12.8843) -> (213.3313, -12.929)
  spline S43 degree 2 poles (213.3313, -12.929) (213.3928, -12.8139) (213.443, -12.6294) (213.4474, -12.5221) knots 0 0 0 1 2 2 2
  spline S44 degree 2 poles (213.4474, -12.5221) (213.4574, -12.2792) (213.1044, -11.9889) (212.7603, -11.9747) knots 0 0 0 1 2 2 2
  spline S45 degree 2 poles (212.7603, -11.9747) (212.4283, -11.9611) (212.0694, -12.1571) (212.0598, -12.3899) knots 0 0 0 1 2 2 2
  spline S46 degree 2 poles (212.0598, -12.3899) (212.0548, -12.5134) (212.1578, -12.7691) (212.2483, -12.8843) knots 0 0 0 1 2 2 2
  spline S47 degree 2 poles (211.6176, -15.5219) (211.6426, -15.0729) (212.1738, -14.6074) (212.639, -14.6333) knots 0 0 0 1 2 2 2
  spline S48 degree 2 poles (212.639, -14.6333) (213.0962, -14.6588) (213.6116, -15.1684) (213.5901, -15.5547) knots 0 0 0 1 2 2 2
  spline S49 degree 2 poles (213.5901, -15.5547) (213.5804, -15.7287) (213.4642, -15.9921) (213.3515, -16.0852) knots 0 0 0 1 2 2 2
  spline S50 degree 2 poles (213.3515, -16.0852) (213.2387, -16.1804) (212.9232, -16.2704) (212.6987, -16.2578) knots 0 0 0 1 2 2 2
  line L26 (212.6987, -16.2578) -> (212.5267, -16.2483)
  line L27 (212.5267, -16.2483) -> (212.599, -14.9517)
  spline S51 degree 2 poles (212.599, -14.9517) (212.2733, -14.9335) (211.9091, -15.2419) (211.8929, -15.5332) knots 0 0 0 1 2 2 2
  spline S52 degree 2 poles (211.8929, -15.5332) (211.8872, -15.6364) (211.9225, -15.8392) (211.9544, -15.9222) knots 0 0 0 1 2 2 2
  spline S53 degree 2 poles (211.9544, -15.9222) (211.9902, -16.0094) (212.0544, -16.1306) (212.0846, -16.1709) knots 0 0 0 1 2 2 2
  line L28 (212.0846, -16.1709) -> (212.0836, -16.1891)
  line L29 (212.0836, -16.1891) -> (211.7398, -16.1699)
  spline S54 degree 2 poles (211.7398, -16.1699) (211.7205, -16.1141) (211.6651, -15.9446) (211.6505, -15.8788) knots 0 0 0 1 2 2 2
  spline S55 degree 2 poles (211.6505, -15.8788) (211.6292, -15.7863) (211.6113, -15.6352) (211.6176, -15.5219) knots 0 0 0 1 2 2 2
  spline S56 degree 2 poles (212.7846, -15.9542) (212.9122, -15.9573) (213.1013, -15.915) (213.1668, -15.868) knots 0 0 0 1 2 2 2
  spline S57 degree 2 poles (213.1668, -15.868) (213.2406, -15.8173) (213.325, -15.6495) (213.3321, -15.5221) knots 0 0 0 1 2 2 2
  spline S58 degree 2 poles (213.3321, -15.5221) (213.3391, -15.3967) (213.2741, -15.2165) (213.2053, -15.1396) knots 0 0 0 1 2 2 2
  spline S59 degree 2 poles (213.2053, -15.1396) (213.1344, -15.0647) (212.9585, -14.9818) (212.8397, -14.9651) knots 0 0 0 1 2 2 2
  line L30 (212.8397, -14.9651) -> (212.7846, -15.9542)
  line L31 (213.7681, -18.7307) -> (213.7692, -18.7146)
  spline S60 degree 2 poles (213.7692, -18.7146) (213.7883, -18.6732) (213.8273, -18.5175) (213.8316, -18.4548) knots 0 0 0 1 2 2 2
  spline S61 degree 2 poles (213.8316, -18.4548) (213.8452, -18.2568) (213.6789, -18.0748) (213.4445, -18.0588) knots 0 0 0 1 2 2 2
  line L32 (213.4445, -18.0588) -> (213.3818, -18.0545)
  line L33 (213.3818, -18.0545) -> (213.3461, -18.576)
  line L34 (213.3461, -18.576) -> (213.0854, -18.5581)
  line L35 (213.0854, -18.5581) -> (213.1204, -18.0467)
  line L36 (213.1204, -18.0467) -> (211.5095, -17.9365)
  line L37 (211.5095, -17.9365) -> (211.5311, -17.6212)
  line L38 (211.5311, -17.6212) -> (213.142, -17.7314)
  line L39 (213.142, -17.7314) -> (213.1565, -17.5192)
  line L40 (213.1565, -17.5192) -> (213.4172, -17.5371)
  line L41 (213.4172, -17.5371) -> (213.4027, -17.7493)
  line L42 (213.4027, -17.7493) -> (213.4654, -17.7536)
  spline S62 degree 2 poles (213.4654, -17.7536) (213.8009, -17.7765) (214.1303, -18.126) (214.1096, -18.4292) knots 0 0 0 1 2 2 2
  spline S63 degree 2 poles (214.1096, -18.4292) (214.1036, -18.5161) (214.0739, -18.6826) (214.0571, -18.7505) knots 0 0 0 1 2 2 2
  line L43 (214.0571, -18.7505) -> (213.7681, -18.7307)
  spline S64 degree 2 poles (211.0685, -19.8661) (211.0518, -19.8972) (210.9973, -20.0168) (210.9727, -20.0941) knots 0 0 0 1 2 2 2
  spline S65 degree 2 poles (210.9727, -20.0941) (210.9435, -20.1791) (210.9052, -20.3244) (210.8982, -20.4112) knots 0 0 0 1 2 2 2
  spline S66 degree 2 poles (210.8982, -20.4112) (210.8863, -20.5566) (210.9466, -20.7647) (211.0107, -20.8269) knots 0 0 0 1 2 2 2
  spline S67 degree 2 poles (211.0107, -20.8269) (211.0749, -20.887) (211.2511, -20.944) (211.3662, -20.9534) knots 0 0 0 1 2 2 2
  line L44 (211.3662, -20.9534) -> (211.5298, -20.9667)
  spline S68 degree 2 poles (211.5298, -20.9667) (211.4291, -20.8304) (211.344, -20.5776) (211.3589, -20.3938) knots 0 0 0 1 2 2 2
  spline S69 degree 2 poles (211.3589, -20.3938) (211.3849, -20.0748) (211.8902, -19.7358) (212.3364, -19.7721) knots 0 0 0 1 2 2 2
  spline S70 degree 2 poles (212.3364, -19.7721) (212.5686, -19.791) (212.9174, -19.9515) (213.0357, -20.0709) knots 0 0 0 1 2 2 2
  spline S71 degree 2 poles (213.0357, -20.0709) (213.1463, -20.1856) (213.2541, -20.485) (213.2416, -20.6385) knots 0 0 0 1 2 2 2
  spline S72 degree 2 poles (213.2416, -20.6385) (213.2297, -20.7839) (213.1438, -20.9903) (213.0725, -21.0923) knots 0 0 0 1 2 2 2
  line L45 (213.0725, -21.0923) -> (213.1498, -21.1168)
  line L46 (213.1498, -21.1168) -> (213.1256, -21.4137)
  line L47 (213.1256, -21.4137) -> (211.4698, -21.2789)
  spline S73 degree 2 poles (211.4698, -21.2789) (210.9933, -21.2401) (210.5828, -20.79) (210.6174, -20.364) knots 0 0 0 1 2 2 2
  spline S74 degree 2 poles (210.6174, -20.364) (210.6286, -20.2266) (210.6964, -19.9435) (210.7427, -19.8233) knots 0 0 0 1 2 2 2
  line L48 (210.7427, -19.8233) -> (211.0699, -19.8499)
  line L49 (211.0699, -19.8499) -> (211.0685, -19.8661)
  line L50 (211.7883, -20.9877) -> (212.8161, -21.0714)
  spline S75 degree 2 poles (212.8161, -21.0714) (212.8821, -20.9589) (212.9467, -20.7649) (212.9548, -20.666) knots 0 0 0 1 2 2 2
  spline S76 degree 2 poles (212.9548, -20.666) (212.9742, -20.4277) (212.6452, -20.1245) (212.316, -20.0977) knots 0 0 0 1 2 2 2
  spline S77 degree 2 poles (212.316, -20.0977) (212.0051, -20.0724) (211.663, -20.2539) (211.644, -20.4882) knots 0 0 0 1 2 2 2
  spline S78 degree 2 poles (211.644, -20.4882) (211.6339, -20.6113) (211.7098, -20.8777) (211.7883, -20.9877) knots 0 0 0 1 2 2 2
  line L51 (210.9793, -24.2532) -> (211.0095, -23.9386)
  line L52 (211.0095, -23.9386) -> (212.0743, -24.0411)
  spline S79 degree 2 poles (212.0743, -24.0411) (212.2034, -24.0535) (212.4275, -24.0506) (212.4976, -24.0207) knots 0 0 0 1 2 2 2
  spline S80 degree 2 poles (212.4976, -24.0207) (212.5718, -23.9892) (212.6536, -23.8587) (212.6649, -23.7417) knots 0 0 0 1 2 2 2
  spline S81 degree 2 poles (212.6649, -23.7417) (212.6761, -23.6247) (212.575, -23.3647) (212.4856, -23.236) knots 0 0 0 1 2 2 2
  line L53 (212.4856, -23.236) -> (211.0901, -23.1017)
  line L54 (211.0901, -23.1017) -> (211.1204, -22.7871)
  line L55 (211.1204, -22.7871) -> (213.7198, -23.0373)
  line L56 (213.7198, -23.0373) -> (213.6895, -23.3519)
  line L57 (213.6895, -23.3519) -> (212.7498, -23.2614)
  spline S82 degree 2 poles (212.7498, -23.2614) (212.8632, -23.4148) (212.9701, -23.6999) (212.9554, -23.8531) knots 0 0 0 1 2 2 2
  spline S83 degree 2 poles (212.9554, -23.8531) (212.929, -24.1274) (212.5361, -24.403) (212.1912, -24.3698) knots 0 0 0 1 2 2 2
  line L58 (212.1912, -24.3698) -> (210.9793, -24.2532)
  line L59 (210.7867, -26.0826) -> (210.8207, -25.7684)
  line L60 (210.8207, -25.7684) -> (212.6858, -25.9705)
  line L61 (212.6858, -25.9705) -> (212.6518, -26.2847)
  line L62 (212.6518, -26.2847) -> (210.7867, -26.0826)
  line L63 (212.9596, -26.3405) -> (212.9982, -25.984)
  line L64 (212.9982, -25.984) -> (213.3245, -26.0193)
  line L65 (213.3245, -26.0193) -> (213.2858, -26.3758)
  line L66 (213.2858, -26.3758) -> (212.9596, -26.3405)
  spline S84 degree 2 poles (210.5019, -28.1114) (210.184, -28.0738) (209.8905, -27.6924) (209.9259, -27.3926) knots 0 0 0 1 2 2 2
  spline S85 degree 2 poles (209.9259, -27.3926) (209.9321, -27.3403) (209.9573, -27.2127) (209.9747, -27.1515) knots 0 0 0 1 2 2 2
  line L67 (209.9747, -27.1515) -> (210.2564, -27.1848)
  line L68 (210.2564, -27.1848) -> (210.2543, -27.2029)
  spline S86 degree 2 poles (210.2543, -27.2029) (210.242, -27.2382) (210.2154, -27.3248) (210.2107, -27.365) knots 0 0 0 1 2 2 2
  spline S87 degree 2 poles (210.2107, -27.365) (210.1959, -27.4898) (210.239, -27.6601) (210.3009, -27.7062) knots 0 0 0 1 2 2 2
  spline S88 degree 2 poles (210.3009, -27.7062) (210.3568, -27.7515) (210.537, -27.7973) (210.6678, -27.8127) knots 0 0 0 1 2 2 2
  line L69 (210.6678, -27.8127) -> (212.1948, -27.9931)
  line L70 (212.1948, -27.9931) -> (212.2345, -27.6571)
  line L71 (212.2345, -27.6571) -> (212.4941, -27.6878)
  line L72 (212.4941, -27.6878) -> (212.4173, -28.3376)
  line L73 (212.4173, -28.3376) -> (210.5019, -28.1114)
  line L74 (212.7269, -28.3762) -> (212.769, -28.0201)
  line L75 (212.769, -28.0201) -> (213.0949, -28.0586)
  line L76 (213.0949, -28.0586) -> (213.0528, -28.4147)
  line L77 (213.0528, -28.4147) -> (212.7269, -28.3762)
  line L78 (210.167, -31.1786) -> (210.2207, -30.7668)
  line L79 (210.2207, -30.7668) -> (211.2087, -30.1927)
  line L80 (211.2087, -30.1927) -> (211.1044, -30.0524)
  line L81 (211.1044, -30.0524) -> (210.3269, -29.9512)
  line L82 (210.3269, -29.9512) -> (210.3677, -29.6378)
  line L83 (210.3677, -29.6378) -> (212.9573, -29.975)
  line L84 (212.9573, -29.975) -> (212.9164, -30.2884)
  line L85 (212.9164, -30.2884) -> (211.4017, -30.0911)
  line L86 (211.4017, -30.0911) -> (212.0914, -30.9287)
  line L87 (212.0914, -30.9287) -> (212.0407, -31.3185)
  line L88 (212.0407, -31.3185) -> (211.3626, -30.4538)
  line L89 (211.3626, -30.4538) -> (210.167, -31.1786)
  line L90 (209.9513, -32.7175) -> (209.9957, -32.4046)
  line L91 (209.9957, -32.4046) -> (212.5813, -32.7715)
  line L92 (212.5813, -32.7715) -> (212.5369, -33.0845)
  line L93 (212.5369, -33.0845) -> (209.9513, -32.7175)
  line L94 (209.4027, -36.341) -> (210.4755, -36.5091)
  spline S89 degree 2 poles (210.4755, -36.5091) (210.6036, -36.5291) (210.8249, -36.5433) (210.8899, -36.5207) knots 0 0 0 1 2 2 2
  spline S90 degree 2 poles (210.8899, -36.5207) (210.961, -36.499) (211.0442, -36.3869) (211.0608, -36.2809) knots 0 0 0 1 2 2 2
  spline S91 degree 2 poles (211.0608, -36.2809) (211.0758, -36.1848) (210.9922, -35.9461) (210.8983, -35.8125) knots 0 0 0 1 2 2 2
  spline S92 degree 2 poles (210.8983, -35.8125) (210.87, -35.8101) (210.7913, -35.8019) (210.7393, -35.7937) knots 0 0 0 1 2 2 2
  line L95 (210.7393, -35.7937) -> (209.5183, -35.6025)
  line L96 (209.5183, -35.6025) -> (209.5672, -35.2902)
  line L97 (209.5672, -35.2902) -> (210.6401, -35.4583)
  spline S93 degree 2 poles (210.6401, -35.4583) (210.7682, -35.4783) (210.9895, -35.4925) (211.0545, -35.4699) knots 0 0 0 1 2 2 2
  spline S94 degree 2 poles (211.0545, -35.4699) (211.1256, -35.4482) (211.2088, -35.3361) (211.2254, -35.2301) knots 0 0 0 1 2 2 2
  spline S95 degree 2 poles (211.2254, -35.2301) (211.2411, -35.13) (211.1498, -34.8881) (211.068, -34.7686) knots 0 0 0 1 2 2 2
  line L98 (211.068, -34.7686) -> (209.6829, -34.5517)
  line L99 (209.6829, -34.5517) -> (209.7318, -34.2394)
  line L100 (209.7318, -34.2394) -> (211.5853, -34.5297)
  line L101 (211.5853, -34.5297) -> (211.5363, -34.842)
  line L102 (211.5363, -34.842) -> (211.3322, -34.81)
  spline S96 degree 2 poles (211.3322, -34.81) (211.4352, -34.9512) (211.5316, -35.2124) (211.5091, -35.3565) knots 0 0 0 1 2 2 2
  spline S97 degree 2 poles (211.5091, -35.3565) (211.4834, -35.5206) (211.2934, -35.7513) (211.113, -35.7907) knots 0 0 0 1 2 2 2
  spline S98 degree 2 poles (211.113, -35.7907) (211.2488, -35.9576) (211.3689, -36.2512) (211.3445, -36.4073) knots 0 0 0 1 2 2 2
  spline S99 degree 2 poles (211.3445, -36.4073) (211.3257, -36.5274) (211.2209, -36.712) (211.1255, -36.7708) knots 0 0 0 1 2 2 2
  spline S100 degree 2 poles (211.1255, -36.7708) (211.0299, -36.8317) (210.7648, -36.8743) (210.5747, -36.8445) knots 0 0 0 1 2 2 2
  line L103 (210.5747, -36.8445) -> (209.3538, -36.6533)
  line L104 (209.3538, -36.6533) -> (209.4027, -36.341)
  line L105 (208.849, -39.6006) -> (208.9032, -39.2893)
  line L106 (208.9032, -39.2893) -> (209.957, -39.4729)
  spline S101 degree 2 poles (209.957, -39.4729) (210.0848, -39.4952) (210.3085, -39.5095) (210.3806, -39.4851) knots 0 0 0 1 2 2 2
  spline S102 degree 2 poles (210.3806, -39.4851) (210.4571, -39.4593) (210.5486, -39.3354) (210.5688, -39.2197) knots 0 0 0 1 2 2 2
  spline S103 degree 2 poles (210.5688, -39.2197) (210.5889, -39.1039) (210.508, -38.8368) (210.4287, -38.7017) knots 0 0 0 1 2 2 2
  line L107 (210.4287, -38.7017) -> (209.0476, -38.461)
  line L108 (209.0476, -38.461) -> (209.1018, -38.1496)
  line L109 (209.1018, -38.1496) -> (210.95, -38.4717)
  line L110 (210.95, -38.4717) -> (210.8957, -38.7831)
  line L111 (210.8957, -38.7831) -> (210.6902, -38.7473)
  spline S104 degree 2 poles (210.6902, -38.7473) (210.7916, -38.9089) (210.8763, -39.2013) (210.8499, -39.353) knots 0 0 0 1 2 2 2
  spline S105 degree 2 poles (210.8499, -39.353) (210.8026, -39.6244) (210.3898, -39.8692) (210.0485, -39.8097) knots 0 0 0 1 2 2 2
  line L112 (210.0485, -39.8097) -> (208.849, -39.6006)
  spline S106 degree 2 poles (209.2119, -42.7829) (208.7461, -42.6947) (208.3234, -42.1506) (208.3942, -41.7764) knots 0 0 0 1 2 2 2
  spline S107 degree 2 poles (208.3942, -41.7764) (208.467, -41.3922) (209.0738, -41.0515) (209.5237, -41.1367) knots 0 0 0 1 2 2 2
  spline S108 degree 2 poles (209.5237, -41.1367) (209.9855, -41.2242) (210.4111, -41.7749) (210.341, -42.1452) knots 0 0 0 1 2 2 2
  spline S109 degree 2 poles (210.341, -42.1452) (210.2701, -42.5194) (209.6757, -42.8707) (209.2119, -42.7829) knots 0 0 0 1 2 2 2
  spline S110 degree 2 poles (209.2726, -42.4624) (209.6309, -42.5303) (210.0286, -42.3355) (210.0743, -42.0946) knots 0 0 0 1 2 2 2
  spline S111 degree 2 poles (210.0743, -42.0946) (210.1199, -41.8538) (209.8213, -41.525) (209.463, -41.4572) knots 0 0 0 1 2 2 2
  spline S112 degree 2 poles (209.463, -41.4572) (209.1147, -41.3912) (208.7066, -41.5861) (208.661, -41.8269) knots 0 0 0 1 2 2 2
  spline S113 degree 2 poles (208.661, -41.8269) (208.6157, -42.0658) (208.9183, -42.3953) (209.2726, -42.4624) knots 0 0 0 1 2 2 2
  spline S114 degree 2 poles (208.6727, -45.7181) (208.2122, -45.6239) (207.7581, -45.0739) (207.8268, -44.7385) knots 0 0 0 1 2 2 2
  spline S115 degree 2 poles (207.8268, -44.7385) (207.8548, -44.6016) (207.9614, -44.4042) (208.0492, -44.3084) knots 0 0 0 1 2 2 2
  line L113 (208.0492, -44.3084) -> (207.2791, -44.1508)
  line L114 (207.2791, -44.1508) -> (207.3424, -43.8412)
  line L115 (207.3424, -43.8412) -> (209.8572, -44.3557)
  line L116 (209.8572, -44.3557) -> (209.7938, -44.6653)
  line L117 (209.7938, -44.6653) -> (209.6013, -44.626)
  spline S116 degree 2 poles (209.6013, -44.626) (209.683, -44.7626) (209.7642, -45.0729) (209.7305, -45.2376) knots 0 0 0 1 2 2 2
  spline S117 degree 2 poles (209.7305, -45.2376) (209.666, -45.5532) (209.0935, -45.8042) (208.6727, -45.7181) knots 0 0 0 1 2 2 2
  spline S118 degree 2 poles (208.7024, -45.3912) (209.018, -45.4558) (209.4063, -45.3264) (209.4522, -45.1021) knots 0 0 0 1 2 2 2
  spline S119 degree 2 poles (209.4522, -45.1021) (209.479, -44.9711) (209.4123, -44.701) (209.3433, -44.5732) knots 0 0 0 1 2 2 2
  line L118 (209.3433, -44.5732) -> (208.2993, -44.3596)
  spline S120 degree 2 poles (208.2993, -44.3596) (208.2169, -44.4689) (208.1379, -44.6326) (208.1152, -44.7438) knots 0 0 0 1 2 2 2
  spline S121 degree 2 poles (208.1152, -44.7438) (208.0661, -44.9839) (208.365, -45.3222) (208.7024, -45.3912) knots 0 0 0 1 2 2 2
  line L119 (206.4275, -48.1515) -> (206.4954, -47.8428)
  line L120 (206.4954, -47.8428) -> (207.37, -48.0352)
  spline S122 degree 2 poles (207.37, -48.0352) (207.2769, -47.8736) (207.2202, -47.5936) (207.2546, -47.4373) knots 0 0 0 1 2 2 2
  spline S123 degree 2 poles (207.2546, -47.4373) (207.3229, -47.1266) (207.9049, -46.8667) (208.3501, -46.9647) knots 0 0 0 1 2 2 2
  spline S124 degree 2 poles (208.3501, -46.9647) (208.5876, -47.0169) (208.9214, -47.2251) (209.0205, -47.359) knots 0 0 0 1 2 2 2
  spline S125 degree 2 poles (209.0205, -47.359) (209.1186, -47.4884) (209.1874, -47.7981) (209.1539, -47.9504) knots 0 0 0 1 2 2 2
  spline S126 degree 2 poles (209.1539, -47.9504) (209.123, -48.0909) (209.0124, -48.2823) (208.9232, -48.3768) knots 0 0 0 1 2 2 2
  line L121 (208.9232, -48.3768) -> (208.998, -48.414)
  line L122 (208.998, -48.414) -> (208.9344, -48.7029)
  line L123 (208.9344, -48.7029) -> (206.4275, -48.1515)
  line L124 (207.6292, -48.0922) -> (208.6739, -48.322)
  spline S127 degree 2 poles (208.6739, -48.322) (208.7569, -48.2179) (208.8425, -48.0458) (208.8655, -47.941) knots 0 0 0 1 2 2 2
  spline S128 degree 2 poles (208.8655, -47.941) (208.9191, -47.6976) (208.6243, -47.3589) (208.2959, -47.2867) knots 0 0 0 1 2 2 2
  spline S129 degree 2 poles (208.2959, -47.2867) (207.9734, -47.2158) (207.581, -47.3493) (207.5322, -47.5709) knots 0 0 0 1 2 2 2
  spline S130 degree 2 poles (207.5322, -47.5709) (207.5039, -47.6995) (207.5608, -47.9693) (207.6292, -48.0922) knots 0 0 0 1 2 2 2
  line L125 (208.0323, -51.1116) -> (208.036, -51.0958)
  spline S131 degree 2 poles (208.036, -51.0958) (208.0541, -51.0626) (208.0761, -50.9866) (208.0885, -50.9333) knots 0 0 0 1 2 2 2